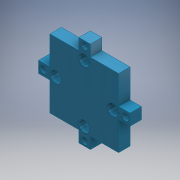
# Autodesk Inventor part: Bottom CLPCLampcell_V5
Saved by Autodesk Inventor 2018 (Build 220112000, 112)
## iProperties
Created: 2018-06-07
Part Number: Bottom CLPCLampcell_V5
Material: Generic
Document SubType Name: Modeling
Designer: Anna Dorfi
Density: 1 g/cm^3
Appearance: Sky Blue Dark
Author: Anna Dorfi
Autodesk Inventor part; units mm, degrees
ref_plane "YZ Plane" through (0, 0, 0) normal (1, 0, 0) x (0, 1, 0)
ref_plane "XZ Plane" through (0, 0, 0) normal (0, 1, 0) x (-1, 0, 0)
ref_plane "XY Plane" through (0, 0, 0) normal (0, 0, 1) x (1, 0, 0)
sketch "Sketch1" plane through (0, 0, 0) normal (0, 1, 0) x (-1, 0, 0)
  circle A0 centre (28.1298, -0.9274) radius 1.5
  circle A1 centre (3.1298, -25.9274) radius 1.5
  circle A2 centre (-21.8702, -0.9274) radius 1.5
  circle A3 centre (3.1298, 24.0726) radius 1.5
  line L0 (33.1298, -30.9274) -> (-26.8702, -30.9274)
  line L1 (-26.8702, -30.9274) -> (-26.8702, 29.0726)
  line L2 (-26.8702, 29.0726) -> (33.1298, 29.0726)
  line L3 (33.1298, 29.0726) -> (33.1298, -30.9274)
  line L4 (33.1298, -30.9274) -> (-26.8702, 29.0726) construction
  line L5 (-26.8702, -30.9274) -> (33.1298, 29.0726) construction
  point P0 (0, 0)
  dimension "d1" = 3
  dimension "d2" = 3
  dimension "d3" = 3
  dimension "d4" = 3
  dimension "d7" = 60
  dimension "d8" = 5
  dimension "d9" = 50
  dimension "d10" = 50
  dimension "d12" = 5
  dimension "d13" = 60
  dimension "d14" = 5
  dimension "d15" = 30
  dimension "d16" = 30
  dimension "d17" = 30
  constraints: 12 end point, 4 centre point, 2 parallel, 1 horizontal, 1 perpendicular
  measures "d1" diameter of A0
  measures "d2" diameter of A1
  measures "d3" diameter of A2
  measures "d4" diameter of A3
  measures "d7" distance of L2.end L0.start
  measures "d8" distance from line of L2 A3.centre
  measures "d9" distance of A3.centre A1.centre
  measures "d10" distance of A0.centre A2.centre
  measures "d12" distance from line of A1.centre L0
  measures "d13" distance of L1.end L2.end
  measures "d14" distance from line of L3 A0.centre
  measures "d15" distance from line of L2 A0.centre
  measures "d16" distance from line of L2 A2.centre
  measures "d17" distance from line of L1 A1.centre
extrude "Extrusion1" add sketch "Sketch1" along normal blind 10
sketch "Sketch2" plane through (0, 10, 0) normal (0, 1, 0) x (1, 0, 0)
  line L0 (26.8702, 30.9274) -> (-33.1298, 30.9274) projected
  line L1 (-7.7791, 30.9274) -> (2.2209, 30.9274)
  line L2 (2.2209, 30.9274) -> (2.2209, 40.9274)
  line L3 (2.2209, 40.9274) -> (-7.7791, 40.9274)
  line L4 (-7.7791, 40.9274) -> (-7.7791, 30.9274)
  line L5 (-33.1298, -29.0726) -> (26.8702, -29.0726) projected
  line L6 (-7.7791, -29.0726) -> (2.2209, -29.0726)
  line L7 (2.2209, -29.0726) -> (2.2209, -39.0726)
  line L8 (2.2209, -39.0726) -> (-7.7791, -39.0726)
  line L9 (-7.7791, -39.0726) -> (-7.7791, -29.0726)
  point P0 (0, 0)
  dimension "d18" = 10
  dimension "d19" = 10
  dimension "d20" = 10
  constraints: 16 end point, 4 parallel, 4 point on line, 2 horizontal, 2 perpendicular
  measures "d18" distance of L3.end L2.end
  measures "d19" distance of L8.end L6.start
  measures "d20" distance of L3.end L1.start
extrude "Extrusion2" add sketch "Sketch2" against normal blind 10
sketch "Sketch3" plane through (0, 10, 0) normal (0, 1, 0) x (1, 0, 0)
  circle A0 centre (-2.7791, 36.9274) radius 2.925
  circle A1 centre (-2.7791, -35.0726) radius 2.925
  line L0 (2.2209, 40.9274) -> (-7.7791, 40.9274) projected
  line L1 (2.2209, -39.0726) -> (-7.7791, -39.0726) projected
  line L2 (-7.7791, 30.9274) -> (-7.7791, 40.9274) projected
  line L3 (-7.7791, -39.0726) -> (-7.7791, -29.0726) projected
  point P0 (0, 0)
  dimension "d23" = 5.85
  dimension "d24" = 5.85
  dimension "d25" = 4
  dimension "d26" = 4
  dimension "d29" = 5
  dimension "d30" = 5
  constraints: 2 centre point
  measures "d23" diameter of A0
  measures "d24" diameter of A1
  measures "d25" distance from line of L0 A0.centre
  measures "d26" distance from line of L1 A1.centre
  measures "d29" distance from line of L2 A0.centre
  measures "d30" distance from line of L3 A1.centre
extrude "Extrusion3" cut sketch "Sketch3" against normal through all
sketch "Sketch4" plane through (0, 0, 0) normal (0, -1, 0) x (1, 0, 0)
  circle A0 centre (-3.1298, 24.0726) radius 1.5 projected
  circle A1 centre (-3.1298, 24.0726) radius 4.75
  circle A2 centre (21.8702, -0.9274) radius 1.5 projected
  circle A3 centre (21.8702, -0.9274) radius 4.75
  circle A4 centre (-3.1298, -25.9274) radius 1.5 projected
  circle A5 centre (-3.1298, -25.9274) radius 4.75
  circle A6 centre (-28.1298, -0.9274) radius 1.5 projected
  circle A7 centre (-28.1298, -0.9274) radius 4.75
  point P0 (0, 0)
  dimension "d31" = 9.5
  dimension "d32" = 9.5
  dimension "d33" = 9.5
  dimension "d34" = 9.5
  constraints: 4 centre point, 4 coincident
  measures "d31" diameter of A1
  measures "d32" diameter of A3
  measures "d33" diameter of A5
  measures "d34" diameter of A7
extrude "Extrusion4" cut sketch "Sketch4" against normal blind 7
sketch "Sketch5" plane through (0, 0, 0) normal (0, -1, 0) x (1, 0, 0)
  line L0 (-33.1298, 29.0726) -> (-33.1298, -30.9274) projected
  line L1 (-33.1298, -5.9274) -> (-43.1298, -5.9274)
  line L2 (-43.1298, -5.9274) -> (-43.1298, 4.0726)
  line L3 (-43.1298, 4.0726) -> (-33.1298, 4.0726)
  line L4 (-33.1298, 4.0726) -> (-33.1298, -5.9274)
  line L5 (-33.1298, -30.9274) -> (-7.7791, -30.9274) projected
  line L6 (26.8702, 29.0726) -> (-33.1298, 29.0726) projected
  line L7 (26.8702, -30.9274) -> (26.8702, 29.0726) projected
  line L8 (26.8702, -5.9274) -> (36.8702, -5.9274)
  line L9 (36.8702, -5.9274) -> (36.8702, 4.0726)
  line L10 (36.8702, 4.0726) -> (26.8702, 4.0726)
  line L11 (26.8702, 4.0726) -> (26.8702, -5.9274)
  line L12 (-33.1298, -30.9274) -> (26.8702, -30.9274) projected
  line L13 (26.8702, 29.0726) -> (2.2209, 29.0726) projected
  point P0 (0, 0)
  point P1 (-7.7791, 29.0726)
  point P2 (2.2209, -30.9274)
  dimension "d37" = 10
  dimension "d38" = 10
  dimension "d39" = 25
  dimension "d40" = 25
  dimension "d41" = 10
  dimension "d42" = 25
  dimension "d43" = 25
  constraints: 16 end point, 4 parallel, 2 horizontal, 2 perpendicular, 2 point on line
  measures "d37" distance of L2.end L3.end
  measures "d38" distance of L1.end L2.end
  measures "d39" distance between parallel lines of L5 L1
  measures "d40" distance between parallel lines of L6 L3
  measures "d41" distance of L10.end L9.end
  measures "d42" distance between parallel lines of L12 L8
  measures "d43" distance between parallel lines of L13 L10
extrude "Extrusion5" add sketch "Sketch5" against normal blind 10 contours L0 L1 L2 L3 | L10 L9 L8 L7
sketch "Sketch6" plane through (0, 0, 0) normal (0, -1, 0) x (1, 0, 0)
  circle A0 centre (-39.1298, -0.9274) radius 2.925
  circle A1 centre (32.8702, -0.9274) radius 2.925
  line L0 (26.8702, -5.9274) -> (36.8702, -5.9274) projected
  line L1 (36.8702, -5.9274) -> (36.8702, 4.0726) projected
  line L2 (-43.1298, -5.9274) -> (-43.1298, 4.0726) projected
  line L3 (-33.1298, -5.9274) -> (-43.1298, -5.9274) projected
  point P0 (0, 0)
  dimension "d46" = 5.85
  dimension "d47" = 5.85
  dimension "d48" = 5
  dimension "d49" = 4
  dimension "d50" = 4
  dimension "d51" = 5
  constraints: 2 centre point
  measures "d46" diameter of A0
  measures "d47" diameter of A1
  measures "d48" distance from line of L0 A1.centre
  measures "d49" distance from line of L1 A1.centre
  measures "d50" distance from line of L2 A0.centre
  measures "d51" distance from line of L3 A0.centre
extrude "Extrusion6" cut sketch "Sketch6" against normal through all
body "Solid1"
